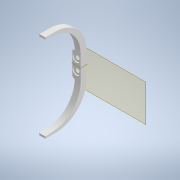
# Autodesk Inventor part: leg
Saved by Autodesk Inventor 2020 (Build 240168000, 168)
## iProperties
Created: 2019-05-07
Part Number: leg
Material: Generic
Document SubType Name: Modeling
Designer: erwin
Density: 1 g/cm^3
Appearance: Default
Author: erwin
Autodesk Inventor part; units mm, degrees
ref_plane "YZ Plane" through (0, 0, 0) normal (1, 0, 0) x (0, 1, 0)
ref_plane "XZ Plane" through (0, 0, 0) normal (0, 1, 0) x (-1, 0, 0)
ref_plane "XY Plane" through (0, 0, 0) normal (0, 0, 1) x (1, 0, 0)
ref_plane "Work Plane1" through (0, 0, 0) normal (0, 0, 1) x (1, 0, 0)
sketch "Sketch1" plane through (0, 0, 0) normal (0, 0, 1) x (1, 0, 0)
  arc A0 (-25.4, 14.25) -> (-27.4, 12.25) centre (-25.4, 12.25) ccw projected
  line L0 (-27.4, 12.25) -> (-27.4, -5.25) projected
  arc A1 (-27.4, -5.25) -> (-25.4, -7.25) centre (-25.4, -5.25) ccw projected
  line L1 (-25.4, -7.25) -> (-20.4, -7.25) projected
  arc A2 (-18.4, -9.25) -> (-20.4, -7.25) centre (-20.4, -9.25) ccw projected
  line L2 (-18.4, -9.25) -> (-18.4, -12.25) projected
  arc A3 (-18.4, -12.25) -> (-16.4, -14.25) centre (-16.4, -12.25) ccw projected
  line L3 (-16.4, -14.25) -> (1.6, -14.25) projected
  arc A4 (1.6, -14.25) -> (3.6, -12.25) centre (1.6, -12.25) ccw projected
  line L4 (3.6, -12.25) -> (3.6, -9.25) projected
  arc A5 (5.6, -7.25) -> (3.6, -9.25) centre (5.6, -9.25) ccw projected
  line L5 (5.6, -7.25) -> (25.4, -7.25) projected
  arc A6 (25.4, -7.25) -> (27.4, -5.25) centre (25.4, -5.25) ccw projected
  line L6 (27.4, -5.25) -> (27.4, 12.25) projected
  arc A7 (27.4, 12.25) -> (25.4, 14.25) centre (25.4, 12.25) ccw projected
  line L7 (25.4, 14.25) -> (20.4, 14.25) projected
  line L8 (20.4, 14.25) -> (20.4, -5.25) projected
  line L9 (20.4, -5.25) -> (1.6, -5.25) projected
  line L10 (1.6, -5.25) -> (1.6, -12.25) projected
  line L11 (1.6, -12.25) -> (-16.4, -12.25) projected
  line L12 (-16.4, -12.25) -> (-16.4, -5.25) projected
  line L13 (-16.4, -5.25) -> (-20.4, -5.25) projected
  line L14 (-20.4, -5.25) -> (-20.4, 14.25) projected
  line L15 (-20.4, 14.25) -> (-25.4, 14.25) projected
  circle A8 centre (24, -0.75) radius 1.25 projected
  circle A9 centre (-24, -0.75) radius 1.25 projected
  circle A10 centre (-24, 8.75) radius 1.25 projected
  circle A11 centre (24, 8.75) radius 1.25 projected
  line L16 (-20.4, -5.25) -> (-20.4, -7.25)
  point P0 (0, 0)
  constraints: 2 end point, 1 vertical
extrude "Extrusion1" add sketch "Sketch1" along normal blind 5 contours L15 L14 L16 L1 A1 L0 A0
ref_plane "Work Plane2" through (-25.4, 3.5, 0) normal (0, -1, 0) x (1, 0, 0)
sketch "Sketch3" plane through (-20.4, -7.25, 0) normal (1, 0, 0) x (0, 0, -1)
  line L0 (0, 19.5) -> (-5, 19.5) projected
  line L1 (0, 21.5) -> (-5, 21.5) projected
  line L2 (0, 21.5) -> (0, 19.5) projected
  arc A0 (0, 21.5) -> (-26.5399, 48.0399) centre (-26.5399, 21.5) ccw
  line L3 (-26.5399, 48.0399) -> (-35, 48.0399)
  line L4 (-35, 48.0399) -> (-35, 46.366)
  line L5 (-35, 46.366) -> (-28.2329, 46.0051)
  arc A1 (-5, 21.5) -> (-28.2329, 46.0051) centre (-29.5399, 21.5) ccw
  line L6 (-5, 0) -> (-5, 21.5) projected
  line L7 (0, 0) -> (0, 21.5) projected
  point P0 (0, 7.25)
  dimension "d9" = 3
  dimension "d12" = 35
  constraints: 6 end point, 4 point on circle, 4 tangent, 2 centre point, 1 perpendicular, 1 vertical
  measures "d9" distance of A0.centre A1.centre
  measures "d12" distance between parallel lines of L2 L4
extrude "Extrusion2" add sketch "Sketch3" against normal blind 5 contours L1 A1 L5 L4 L3 A0
sketch "Sketch2" plane through (0, 0, 5) normal (0, 0, 1) x (1, 0, 0)
  circle A0 centre (-24, -0.75) radius 1.25 projected
  circle A1 centre (-24, 8.75) radius 1.25 projected
  point P0 (0, 0)
  constraints: 2 coincident
hole "Hole1" at (-24, -0.75, 5) at (-24, 8.75, 5) direction (0, 0, -1) diameter 3.2 end through all counterbore diameter 6.5 counterbore depth 1
mirror "Mirror1" about plane through (-25.4, 3.5, 0) normal (0, -1, 0) of "Extrusion2"
body "Solid1"
